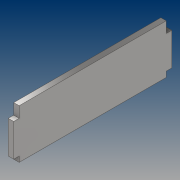
# Autodesk Inventor part: 03_Tam_top_vs_bottom
Saved by Autodesk Inventor 2021 (Build 250183000, 183)
## iProperties
Created: 2024-04-07
Part Number: 03_Tam_top_vs_bottom
Material: Stainless Steel, Austenitic
Document SubType Name: Modeling
Designer: Admin
Density: 8 g/cm^3
Appearance: Semi-Polished
Mass: 1944 g
Surface Area: 558 cm^2
Volume: 243 cm^3
Author: Admin
Autodesk Inventor part; units mm, degrees
ref_plane "YZ Plane" through (0, 0, 0) normal (1, 0, 0) x (0, 1, 0)
ref_plane "XZ Plane" through (0, 0, 0) normal (0, 1, 0) x (-1, 0, 0)
ref_plane "XY Plane" through (0, 0, 0) normal (0, 0, 1) x (1, 0, 0)
sketch "Sketch1" plane through (0, 0, 0) normal (1, 0, 0) x (0, 1, 0)
  line L0 (-45, 135) -> (45, 135)
  line L1 (45, 135) -> (45, -135)
  line L2 (45, -135) -> (-45, -135)
  line L3 (-45, -135) -> (-45, 135)
  line L4 (-45, 135) -> (45, -135) construction
  line L5 (45, 135) -> (-45, -135) construction
  point P0 (0, 0)
  dimension "d0" = 90
  dimension "d1" = 270
  constraints: 12 end point, 2 midpoint, 2 parallel, 1 horizontal, 1 perpendicular
  measures "d0" distance of L1.end L2.end
  measures "d1" distance of L0.end L1.end
extrude "Extrusion1" add sketch "Sketch1" along normal blind 10
sketch "Sketch2" plane through (0, 0, 0) normal (-1, 0, 0) x (0, 0, 1)
  line L0 (-135, -45) -> (-135, 45) projected
  line L1 (135, -45) -> (-135, -45) projected
  line L2 (135, 45) -> (135, -45) projected
  line L3 (-135, 45) -> (135, 45) projected
  line L4 (0, 45) -> (0, -5)
  line L5 (145, 25) -> (-145, 25)
  line L6 (-145, 25) -> (-145, -35)
  line L7 (-145, -35) -> (145, -35)
  line L8 (145, -35) -> (145, 25)
  line L9 (145, 25) -> (-145, -35) construction
  line L10 (-145, 25) -> (145, -35) construction
  point P0 (-135, -35)
  point P1 (-135, 25)
  point P2 (135, 25)
  point P3 (135, -35)
  dimension "d8" = 90
  dimension "d9" = 50
  dimension "d10" = 60
  dimension "d11" = 290
  dimension "d12" = 270
  constraints: 14 end point, 3 midpoint, 2 parallel, 1 horizontal, 1 perpendicular, 1 vertical
  measures "d8" distance of L0.start L0.end
  measures "d9" distance of L4.start L4.end
  measures "d10" distance of L5.end L6.end
  measures "d11" distance of L6.end L7.end
  measures "d12" distance of L1.start L0.start
extrude "Extrusion2" add sketch "Sketch2" against normal blind 10 contours L7 L6 L5 L0 | L2 L5 L8 L7
body "Solid1"
